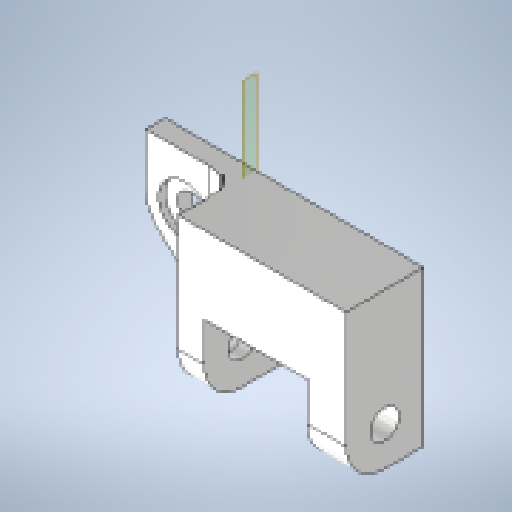
# Autodesk Inventor part: Mod Mount
Saved by Autodesk Inventor 2023.2 (Build 272271000, 271)
## iProperties
Created: 2024-04-01
Part Number: Mod Mount
Material: UHMW, White
Document SubType Name: Modeling
Designer: Nathan Cai
Mass: 23.2616 g
Surface Area: 81.0979 cm^2
Volume: 24.7463 cm^3
Density: 0.94 g/cm^3
Appearance: Smooth - White
Author: Nathan Cai
Autodesk Inventor part; units mm, degrees
ref_plane "YZ Plane" through (0, 0, 0) normal (1, 0, 0) x (0, 1, 0)
ref_plane "XZ Plane" through (0, 0, 0) normal (0, 1, 0) x (-1, 0, 0)
ref_plane "XY Plane" through (0, 0, 0) normal (0, 0, 1) x (1, 0, 0)
sketch "Sketch18" plane through (0, 0, 0) normal (0, 0, 1) x (1, 0, 0)
  circle A0 centre (0, 0) radius 3.302
  circle A1 centre (0, 0) radius 9.525
  line L0 (-9.525, -22.225) -> (53.975, -22.225)
  line L1 (53.975, -22.225) -> (53.975, 9.525)
  line L2 (53.975, 9.525) -> (-9.525, 9.525)
  line L3 (-9.525, 9.525) -> (-9.525, -22.225)
  dimension "d100" = 6.604
  dimension "d101" = 19.05
  dimension "d102" = 63.5
  dimension "d103" = 31.75
  constraints: 8 end point, 2 centre point, 2 coincident, 2 parallel, 2 tangent, 1 horizontal, 1 perpendicular
  measures "d100" diameter of A0
  measures "d101" diameter of A1
  measures "d102" distance of L2.end L1.end
  measures "d103" distance of L1.end L0.end
extrude "Extrusion17" add sketch "Sketch18" along normal blind 19.05
sketch "Sketch19" plane through (-9.525, -22.225, 0) normal (-1, 0, 0) x (0, 0, 1)
  circle A0 centre (9.525, 9.525) radius 9.525 construction
  circle A1 centre (9.525, 9.525) radius 3.556
  line L0 (0, 31.75) -> (0, 0) projected
  line L1 (0, 0) -> (19.05, 0) projected
  point P0 (0, 22.225)
  dimension "d106" = 19.05
  dimension "d107" = 7.112
  constraints: 2 centre point, 2 tangent, 1 coincident
  measures "d106" diameter of A0
  measures "d107" diameter of A1
extrude "Extrusion18" cut sketch "Sketch19" against normal through all
sketch "Sketch20" plane through (0, 0, 19.05) normal (0, 0, 1) x (1, 0, 0)
  line L0 (12.7, -41.275) -> (38.1, -41.275)
  line L1 (38.1, -41.275) -> (38.1, -3.175)
  line L2 (38.1, -3.175) -> (12.7, -3.175)
  line L3 (12.7, -3.175) -> (12.7, -41.275)
  line L4 (-9.525, -22.225) -> (53.975, -22.225) projected
  line L5 (12.7, -41.275) -> (38.1, -3.175) construction
  line L6 (38.1, -41.275) -> (12.7, -3.175) construction
  circle A0 centre (0, 0) radius 3.302 projected
  point P0 (25.4, -22.225)
  point P1 (12.7, -22.225)
  point P2 (38.1, -22.225)
  dimension "d110" = 25.4
  dimension "d111" = 38.1
  dimension "d112" = 12.7
  constraints: 12 end point, 2 midpoint, 2 parallel, 1 horizontal, 1 perpendicular, 1 point on line
  measures "d110" distance of L2.end L1.end
  measures "d111" distance of L1.end L0.end
  measures "d112" distance from line of A0.centre L3
extrude "Extrusion19" cut sketch "Sketch20" against normal through all contours L3 L2 L1 L4
sketch "Sketch21" plane through (-9.525, -22.225, 0) normal (-1, 0, 0) x (0, 0, 1)
  circle A0 centre (9.525, 9.525) radius 3.556 projected
  circle A1 centre (9.525, 9.525) radius 6.35
  line L0 (3.175, -9.525) -> (15.875, -9.525)
  line L1 (15.875, -9.525) -> (15.875, 9.525)
  line L2 (15.875, 9.525) -> (3.175, 9.525) construction
  line L3 (3.175, 9.525) -> (3.175, -9.525)
  line L4 (19.05, 0) -> (0, 0) projected
  line L5 (3.175, -9.525) -> (15.875, 9.525) construction
  line L6 (15.875, -9.525) -> (3.175, 9.525) construction
  point P0 (0, 22.225)
  point P1 (9.525, 0)
  point P2 (3.175, 0)
  point P3 (15.875, 0)
  point P4 (3.175, 9.525)
  dimension "d115" = 12.7
  constraints: 12 end point, 3 midpoint, 2 parallel, 2 vertical, 1 coincident, 1 horizontal, 1 perpendicular, 3 other
extrude "Extrusion20" cut sketch "Sketch21" against normal blind 19.05 contours A1
sketch "Sketch22" plane through (0, 0, 19.05) normal (0, 0, 1) x (1, 0, 0)
  circle A0 centre (0, 0) radius 9.525
  line L0 (-9.525, 9.525) -> (-9.525, -22.225) projected
  line L1 (9.525, -22.225) -> (-9.525, -22.225) projected
  line L2 (9.525, -22.225) -> (-6.569, -6.8974)
  line L3 (12.7, -22.225) -> (12.7, -3.175) projected
  line L4 (53.975, 9.525) -> (-9.525, 9.525) projected
  point P0 (-9.525, 0)
  point P1 (0, 9.525)
  dimension "d118" = 3.175
  constraints: 2 end point, 1 coincident, 1 point on line, 1 vertical, 4 other
  measures "d118" distance from line of L3 L2.start
extrude "Extrusion21" cut sketch "Sketch22" against normal through all contours L2 L1 L0 A0 | L0 L4 A0
fillet "Fillet12" radius 1.5875 1 edges at (9.525, -12.7, 3.175)
fillet "Fillet13" radius 9.525 4 edges at (11.1125, -22.225, 19.05) (11.1125, -22.225, 0) (46.0375, -22.225, 19.05) (46.0375, -22.225, 0)
sketch "Sketch25" plane through (53.975, 9.525, 19.05) normal (1, 0, 0) x (0, 0, -1)
  line L0 (0, -22.225) -> (0, -12.7) projected
  line L1 (0, -12.7) -> (12.7, 0)
  line L2 (19.05, 0) -> (0, 0) projected
  line L3 (0, -22.225) -> (0, 0) projected
  point P0 (19.05, -9.525)
  dimension "d131" = 6.35
  constraints: 2 end point, 1 point on line
  measures "d131" distance of L2.start L1.end
extrude "Extrusion24" cut sketch "Sketch25" against normal through all
sketch "Sketch26" plane through (0, 0, 19.05) normal (0, 0, 1) x (1, 0, 0)
  circle A0 centre (0, 0) radius 6.35
  dimension "d134" = 12.7
  constraints: 1 centre point, 1 coincident
  measures "d134" diameter of A0
extrude "Extrusion25" cut sketch "Sketch26" against normal blind 15.875
fillet "Fillet16" radius 3.175 1 edges at (25.4, -3.175, 19.05)
fillet "Fillet17" radius 6.35 3 edges at (9.0996, -3.175, 19.05) (-7.2398, -3.175, 19.05) (46.0375, -3.175, 19.05)
fillet "Fillet18" radius 1.5875 1 edges at (-6.35, 0, 3.175)
body "Solid2"
